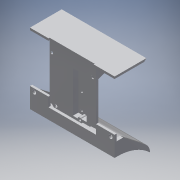
# Autodesk Inventor part: Chasis_base
Saved by Autodesk Inventor 2017 (Build 210142000, 142)
## iProperties
Created: 2018-02-27
Part Number: Chasis_base
Material: PAEK Plastic
Document SubType Name: Modeling
Designer: bradl
Density: 1.32 g/cm^3
Appearance: Smooth - White
Author: bradl
Autodesk Inventor part; units mm, degrees
ref_plane "YZ Plane" through (0, 0, 0) normal (1, 0, 0) x (0, 1, 0)
ref_plane "XZ Plane" through (0, 0, 0) normal (0, 1, 0) x (-1, 0, 0)
ref_plane "XY Plane" through (0, 0, 0) normal (0, 0, 1) x (1, 0, 0)
sketch "Sketch1" plane through (0, 0, 0) normal (0, 0, 1) x (1, 0, 0)
  arc A0 (-11.1125, -2.3813) -> (-3.175, -2.3812) centre (-7.1437, -2.3813) ccw projected
  arc A1 (5.2705, 38.0653) -> (-2.667, 38.0653) centre (1.3018, 38.0653) ccw projected
  line L0 (1.3018, 42.034) -> (-11.1125, 42.034)
  line L1 (-11.1125, 42.034) -> (-11.1125, -6.35)
  line L2 (-11.1125, -6.35) -> (5.2705, -6.35)
  line L3 (5.2705, -6.35) -> (5.2705, 42.034)
  line L4 (5.2705, 42.034) -> (1.3018, 42.034)
  circle A2 centre (-7.1437, -2.3813) radius 1.27 projected
  circle A3 centre (-7.1438, 16.9213) radius 1.27 projected
  circle A4 centre (1.3018, 18.7628) radius 1.27 projected
  circle A5 centre (1.3018, 38.0653) radius 1.27 projected
  circle A6 centre (-7.1437, -2.3813) radius 1.27
  circle A7 centre (-7.1438, 16.9213) radius 1.27
  circle A8 centre (1.3018, 18.7628) radius 1.27
  circle A9 centre (1.3018, 38.0653) radius 1.27
  point P0 (0, 0)
  constraints: 10 end point, 4 centre point, 4 coincident, 4 concentric, 4 perpendicular, 1 horizontal, 1 point on circle, 1 point on line, 1 tangent
extrude "Extrusion1" add sketch "Sketch1" along normal blind 2.54
sketch "Sketch2" plane through (0, 0, 2.54) normal (0, 0, 1) x (1, 0, 0)
  circle A0 centre (1.3018, 38.0653) radius 1.27 projected
  circle A1 centre (1.3018, 18.7628) radius 1.27 projected
  circle A2 centre (-7.1438, 16.9213) radius 1.27 projected
  circle A3 centre (-7.1437, -2.3813) radius 1.27 projected
  line L0 (5.2705, 42.034) -> (-11.1125, 42.034) projected
  line L1 (-11.1125, 42.034) -> (-11.1125, -6.35) projected
  line L2 (-11.1125, -6.35) -> (5.2705, -6.35) projected
  line L3 (5.2705, -6.35) -> (5.2705, 42.034) projected
  line L4 (-11.1125, -6.35) -> (5.2705, -6.35) projected
  line L5 (5.2705, -6.35) -> (5.2705, 42.034) projected
  line L6 (5.2705, -6.35) -> (5.2705, 42.034)
  line L7 (5.2705, 42.034) -> (-11.1125, 42.034) projected
  line L8 (5.2705, 42.034) -> (-11.1125, 42.034)
  line L9 (-11.1125, 42.034) -> (-11.1125, -6.35) projected
  line L10 (-11.1125, 42.034) -> (-11.1125, -6.35)
  line L11 (-11.1125, -6.35) -> (5.2705, -6.35)
  line L12 (5.2705, -6.35) -> (5.2705, -8.89) construction
  line L13 (-11.1125, -6.35) -> (-13.6525, -6.35) construction
  line L14 (5.2705, -8.89) -> (-13.6525, -8.89)
  line L15 (-11.1125, 42.034) -> (-11.1125, 44.574) construction
  line L16 (5.2705, 42.034) -> (7.8105, 42.034) construction
  line L17 (-13.6525, -8.89) -> (-13.6525, 44.574)
  line L18 (-13.6525, 44.574) -> (7.8105, 44.574)
  line L19 (7.8105, 44.574) -> (7.8105, -8.89)
  line L20 (7.8105, -8.89) -> (5.2705, -8.89)
  point P0 (0, 0)
  dimension "d2" = 2.54
  dimension "d3" = 2.54
  dimension "d4" = 2.54
  dimension "d5" = 2.54
  constraints: 26 end point, 4 collinear, 3 perpendicular, 2 horizontal, 2 point on line, 2 vertical
  measures "d2" distance of L2.end L12.end
  measures "d3" distance of L1.end L13.end
  measures "d4" distance of L0.end L15.end
  measures "d5" distance of L0.start L16.end
extrude "Extrusion2" add sketch "Sketch2" along normal blind 5.08 and the other way blind 2.54 contours L14 L17 L18 L19 L20
sketch "Sketch3" plane through (0, 0, 7.62) normal (0, 0, 1) x (1, 0, 0)
  line L0 (7.8105, -8.89) -> (7.8105, 44.574) projected
  line L1 (-13.6525, -8.89) -> (7.8105, -8.89) projected
  line L2 (-13.6525, 44.574) -> (-13.6525, -8.89) projected
  line L3 (7.8105, 44.574) -> (-13.6525, 44.574) projected
  line L4 (-13.6525, 44.574) -> (7.8105, 44.574) projected
  line L5 (7.8105, 44.574) -> (-13.6525, 44.574)
  line L6 (-13.6525, 44.574) -> (-13.6525, -8.89)
  line L7 (-13.6525, -8.89) -> (7.8105, -8.89)
  line L8 (7.8105, -8.89) -> (7.8105, 44.574)
  line L9 (20.033, 8.7532) -> (20.033, 11.6691) projected
  line L10 (-41.2425, 9.6344) -> (-41.2425, 7.0138) projected
  line L11 (20.033, 8.7532) -> (17.493, 8.7532) construction
  line L12 (-41.2425, 7.0138) -> (-38.7025, 7.0138) construction
  line L13 (17.493, 8.7532) -> (-38.7025, 8.7532) construction
  line L14 (17.493, 8.7532) -> (17.493, 59.5532) construction
  line L15 (17.493, 59.5532) -> (-38.7025, 59.5532) construction
  line L16 (-38.7025, 59.5532) -> (-38.7025, -39.5068) construction
  line L17 (-38.7025, -39.5068) -> (17.493, -39.5068) construction
  line L18 (17.493, -39.5068) -> (17.493, 8.7532) construction
  line L19 (17.493, 59.5532) -> (-38.7025, 59.5532)
  line L20 (-38.7025, 59.5532) -> (-38.7025, -39.5068)
  line L21 (-38.7025, -39.5068) -> (17.493, -39.5068)
  line L22 (17.493, -39.5068) -> (17.493, 59.5532)
  line L23 (-11.1125, 42.034) -> (5.2705, 42.034) projected
  line L24 (-11.1125, 42.034) -> (-11.1125, -6.35) projected
  line L25 (5.2705, 42.034) -> (-11.1125, 42.034)
  line L26 (-11.1125, 42.034) -> (-11.1125, -6.35)
  line L27 (-11.1125, -6.35) -> (5.2705, -6.35)
  line L28 (5.2705, -6.35) -> (5.2705, 42.034)
  point P0 (0, 0)
  dimension "d10" = 2.54
  dimension "d11" = 2.54
  dimension "d12" = 50.8
  dimension "d13" = 99.06
  constraints: 40 end point, 6 horizontal, 6 parallel, 6 perpendicular, 1 collinear, 1 point on line, 1 vertical
  measures "d10" distance of L9.start L11.end
  measures "d11" distance of L10.end L12.end
  measures "d12" distance of L11.end L14.end
  measures "d13" distance of L15.end L16.end
extrude "Extrusion3" add sketch "Sketch3" along normal blind 2.54 contours L1 L2 L3 L0 | L22 L21 L20 L19
sketch "Sketch4" plane through (0, 0, 7.62) normal (0, 0, -1) x (-1, 0, 0)
  line L0 (18.4925, 33.414) -> (14.6525, 33.414)
  line L1 (18.4925, 33.414) -> (18.4925, 23.414) projected
  line L2 (14.6525, 23.414) -> (14.6525, 33.414) projected
  line L3 (18.4925, 23.414) -> (14.6525, 23.414)
  line L4 (31.1925, 23.414) -> (31.1925, 33.414) projected
  line L5 (35.0325, 33.414) -> (31.1925, 33.414)
  line L6 (35.0325, 33.414) -> (35.0325, 23.414) projected
  line L7 (35.0325, 23.414) -> (31.1925, 23.414)
  line L8 (14.6525, 23.414) -> (18.4925, 23.414)
  line L9 (18.4925, 23.414) -> (18.4925, 33.414)
  line L10 (18.4925, 33.414) -> (14.6525, 33.414)
  line L11 (14.6525, 33.414) -> (14.6525, 23.414)
  line L12 (31.1925, 23.414) -> (35.0325, 23.414)
  line L13 (35.0325, 23.414) -> (35.0325, 33.414)
  line L14 (35.0325, 33.414) -> (31.1925, 33.414)
  line L15 (31.1925, 33.414) -> (31.1925, 23.414)
  point P0 (0, 0)
  constraints: 24 end point, 6 horizontal, 4 parallel, 2 perpendicular, 3 other
extrude "Extrusion4" add sketch "Sketch4" along normal blind 12.7
sketch "Sketch5" plane through (-35.0325, 23.414, 7.62) normal (-1, 0, 0) x (0, 0, 1)
  line L0 (0, 0) -> (-12.7, 0) projected
  line L1 (0, 10) -> (-12.7, 10) projected
  circle A0 centre (-12.7, 5.0827) radius 4.9173
  point P0 (-7.62, -23.414)
  constraints: 1 vertical alignment, 2 other
extrude "Extrusion5" cut sketch "Sketch5" against normal blind 20.6375
sketch "Sketch6" plane through (17.493, -39.5068, 7.62) normal (1, 0, 0) x (0, 0, -1)
  line L0 (0, 0) -> (0, 99.06) projected
  line L1 (0, 99.06) -> (0, 15.8755) construction
  line L2 (-13.9711, 65.9208) -> (-12.7011, 65.9208) construction
  arc A0 (-12.7011, 65.9208) -> (-12.403, 63.5609) centre (12.62, 67.9208) ccw construction
  line L3 (-12.403, 63.5609) -> (-13.6331, 63.245) construction
  line L4 (-13.6331, 63.245) -> (-12.6383, 59.3707) construction
  line L5 (-12.6383, 59.3707) -> (-11.4082, 59.6865) construction
  arc A1 (-11.4082, 59.6865) -> (-10.5326, 57.4749) centre (12.62, 67.9208) ccw construction
  line L6 (-10.5326, 57.4749) -> (-11.6455, 56.8631) construction
  line L7 (-11.6455, 56.8631) -> (-9.7185, 53.3578) construction
  line L8 (-9.7185, 53.3578) -> (-8.6056, 53.9697) construction
  arc A2 (-8.6056, 53.9697) -> (-7.2074, 52.0452) centre (12.62, 67.9208) ccw construction
  line L9 (-7.2074, 52.0452) -> (-8.1332, 51.1759) construction
  line L10 (-8.1332, 51.1759) -> (-5.395, 48.26) construction
  line L11 (-5.395, 48.26) -> (-4.4692, 49.1294) construction
  arc A3 (-4.4692, 49.1294) -> (-2.6364, 47.6131) centre (12.62, 67.9208) ccw construction
  line L12 (-2.6364, 47.6131) -> (-3.3169, 46.5408) construction
  line L13 (-3.3169, 46.5408) -> (0.0604, 44.3975) construction
  line L14 (0.0604, 44.3975) -> (0.7409, 45.4698) construction
  arc A4 (0.7409, 45.4698) -> (2.8932, 44.457) centre (12.62, 67.9208) ccw construction
  line L15 (2.8932, 44.457) -> (2.5008, 43.2492) construction
  line L16 (2.5008, 43.2492) -> (6.305, 42.0131) construction
  line L17 (6.305, 42.0131) -> (6.6975, 43.221) construction
  arc A5 (6.6975, 43.221) -> (9.034, 42.7752) centre (12.62, 67.9208) ccw construction
  line L18 (9.034, 42.7752) -> (8.9543, 41.5077) construction
  line L19 (8.9543, 41.5077) -> (12.9464, 41.2566) construction
  line L20 (12.9464, 41.2566) -> (13.0261, 42.5241) construction
  arc A6 (13.0261, 42.5241) -> (15.4001, 42.6734) centre (12.62, 67.9208) ccw construction
  line L21 (15.4001, 42.6734) -> (15.6381, 41.4259) construction
  line L22 (15.6381, 41.4259) -> (19.5673, 42.1755) construction
  line L23 (19.5673, 42.1755) -> (19.3293, 43.423) construction
  arc A7 (19.3293, 43.423) -> (21.5916, 44.158) centre (12.62, 67.9208) ccw construction
  line L24 (21.5916, 44.158) -> (22.1323, 43.0089) construction
  line L25 (22.1323, 43.0089) -> (25.7516, 44.712) construction
  line L26 (25.7516, 44.712) -> (25.2109, 45.8611) construction
  arc A8 (25.2109, 45.8611) -> (27.2193, 47.1357) centre (12.62, 67.9208) ccw construction
  line L27 (27.2193, 47.1357) -> (28.0288, 46.1572) construction
  line L28 (28.0288, 46.1572) -> (31.1109, 48.7068) construction
  line L29 (31.1109, 48.7068) -> (30.3013, 49.6854) construction
  arc A9 (30.3013, 49.6854) -> (31.9297, 51.4194) centre (12.62, 67.9208) ccw construction
  line L30 (31.9297, 51.4194) -> (32.9571, 50.6729) construction
  line L31 (32.9571, 50.6729) -> (35.3083, 53.909) construction
  line L32 (35.3083, 53.909) -> (34.2808, 54.6555) construction
  arc A10 (34.2808, 54.6555) -> (35.4267, 56.7399) centre (12.62, 67.9208) ccw construction
  line L33 (35.4267, 56.7399) -> (36.6076, 56.2724) construction
  line L34 (36.6076, 56.2724) -> (38.0801, 59.9915) construction
  line L35 (38.0801, 59.9915) -> (36.8992, 60.459) construction
  arc A11 (36.8992, 60.459) -> (37.4908, 62.763) centre (12.62, 67.9208) ccw construction
  line L36 (37.4908, 62.763) -> (38.7508, 62.6038) construction
  line L37 (38.7508, 62.6038) -> (39.2521, 66.5723) construction
  line L38 (39.2521, 66.5723) -> (37.9921, 66.7315) construction
  arc A12 (37.9921, 66.7315) -> (37.9921, 69.1102) centre (12.62, 67.9208) ccw construction
  line L39 (37.9921, 69.1102) -> (39.2521, 69.2693) construction
  line L40 (39.2521, 69.2693) -> (38.7508, 73.2378) construction
  line L41 (38.7508, 73.2378) -> (37.4908, 73.0786) construction
  arc A13 (37.4908, 73.0786) -> (36.8992, 75.3826) centre (12.62, 67.9208) ccw construction
  line L42 (36.8992, 75.3826) -> (38.0801, 75.8501) construction
  line L43 (38.0801, 75.8501) -> (36.6076, 79.5692) construction
  line L44 (36.6076, 79.5692) -> (35.4267, 79.1017) construction
  arc A14 (35.4267, 79.1017) -> (34.2808, 81.1862) centre (12.62, 67.9208) ccw construction
  line L45 (34.2808, 81.1862) -> (35.3083, 81.9327) construction
  line L46 (35.3083, 81.9327) -> (32.9571, 85.1687) construction
  line L47 (32.9571, 85.1687) -> (31.9297, 84.4222) construction
  arc A15 (31.9297, 84.4222) -> (30.3013, 86.1562) centre (12.62, 67.9208) ccw construction
  line L48 (30.3013, 86.1562) -> (31.1109, 87.1348) construction
  line L49 (31.1109, 87.1348) -> (28.0288, 89.6845) construction
  line L50 (28.0288, 89.6845) -> (27.2193, 88.7059) construction
  arc A16 (27.2193, 88.7059) -> (25.2109, 89.9805) centre (12.62, 67.9208) ccw construction
  line L51 (25.2109, 89.9805) -> (25.7516, 91.1296) construction
  line L52 (25.7516, 91.1296) -> (22.1323, 92.8328) construction
  line L53 (22.1323, 92.8328) -> (21.5916, 91.6836) construction
  arc A17 (21.5916, 91.6836) -> (19.3293, 92.4187) centre (12.62, 67.9208) ccw construction
  line L54 (19.3293, 92.4187) -> (19.5673, 93.6662) construction
  line L55 (19.5673, 93.6662) -> (15.6381, 94.4157) construction
  line L56 (15.6381, 94.4157) -> (15.4001, 93.1682) construction
  arc A18 (15.4001, 93.1682) -> (13.0261, 93.3176) centre (12.62, 67.9208) ccw construction
  line L57 (13.0261, 93.3176) -> (12.9464, 94.5851) construction
  line L58 (12.9464, 94.5851) -> (8.9543, 94.3339) construction
  line L59 (8.9543, 94.3339) -> (9.034, 93.0664) construction
  arc A19 (9.034, 93.0664) -> (6.6975, 92.6207) centre (12.62, 67.9208) ccw construction
  line L60 (6.6975, 92.6207) -> (6.305, 93.8285) construction
  line L61 (6.305, 93.8285) -> (2.5008, 92.5925) construction
  line L62 (2.5008, 92.5925) -> (2.8932, 91.3846) construction
  arc A20 (2.8932, 91.3846) -> (0.7409, 90.3718) centre (12.62, 67.9208) ccw construction
  line L63 (0.7409, 90.3718) -> (0.0604, 91.4441) construction
  line L64 (0.0604, 91.4441) -> (-3.3169, 89.3008) construction
  line L65 (-3.3169, 89.3008) -> (-2.6364, 88.2285) construction
  arc A21 (-2.6364, 88.2285) -> (-4.4692, 86.7123) centre (12.62, 67.9208) ccw construction
  line L66 (-4.4692, 86.7123) -> (-5.395, 87.5816) construction
  line L67 (-5.395, 87.5816) -> (-8.1332, 84.6658) construction
  line L68 (-8.1332, 84.6658) -> (-7.2074, 83.7964) construction
  arc A22 (-7.2074, 83.7964) -> (-8.6056, 81.872) centre (12.62, 67.9208) ccw construction
  line L69 (-8.6056, 81.872) -> (-9.7185, 82.4838) construction
  line L70 (-9.7185, 82.4838) -> (-11.6455, 78.9786) construction
  line L71 (-11.6455, 78.9786) -> (-10.5326, 78.3668) construction
  arc A23 (-10.5326, 78.3668) -> (-11.4082, 76.1551) centre (12.62, 67.9208) ccw construction
  line L72 (-11.4082, 76.1551) -> (-12.6383, 76.4709) construction
  line L73 (-12.6383, 76.4709) -> (-13.6331, 72.5966) construction
  line L74 (-13.6331, 72.5966) -> (-12.403, 72.2808) construction
  arc A24 (-12.403, 72.2808) -> (-12.7011, 69.9208) centre (12.62, 67.9208) ccw construction
  line L75 (-12.7011, 69.9208) -> (-13.9711, 69.9208) construction
  line L76 (-13.9711, 69.9208) -> (-13.9711, 65.9208) construction
  circle A25 centre (12.62, 67.9208) radius 21.59 construction
  circle A26 centre (12.62, 67.9208) radius 26.6867 construction
  line L77 (0, 99.06) -> (39.3067, 99.06) construction
  line L78 (39.3067, 99.06) -> (39.3067, 0.6575) construction
  arc A27 (39.3067, 0.6575) -> (0, 15.8755) centre (0.9026, -40.1652) ccw
  line L79 (39.3067, 0.6575) -> (39.3067, 7.6204)
  line L80 (39.3067, 0.6575) -> (46.2696, 0.6575) construction
  line L81 (0, 99.06) -> (0, 0) projected
  arc A28 (39.3067, 7.6204) -> (0, 20.9929) centre (1.7012, -38.4614) ccw
  line L82 (0, 20.9929) -> (0, 15.8755)
  line L83 (0, 20.9929) -> (5.1174, 20.9929) construction
  point P0 (7.62, 39.5068)
  dimension "d20" = 90
  dimension "d21" = 90
  dimension "d22" = 90
  constraints: 14 end point, 4 point on circle, 3 centre point, 3 horizontal, 2 perpendicular, 2 point on line, 1 coincident, 1 vertical
  measures "d20" angle of L77 L78
  measures "d21" angle of L80 L79
  measures "d22" angle of L82 L83
extrude "Extrusion6" add sketch "Sketch6" against normal blind 56.1848
sketch "Sketch7" plane through (-38.7025, -39.5068, 7.62) normal (-1, 0, 0) x (0, 0, 1)
  arc A0 (0, 15.8755) -> (-39.3067, 0.6575) centre (-0.9026, -40.1652) ccw projected
  line L0 (0, 99.06) -> (0, 0) projected
  line L1 (0, 0) -> (2.54, 0) projected
  line L2 (2.54, 99.06) -> (2.54, 0) projected
  line L3 (0, 99.06) -> (2.54, 99.06) projected
  line L4 (0, 15.8755) -> (0, 0)
  line L5 (0, 0) -> (2.54, 0) projected
  line L6 (2.54, 0) -> (2.54, 15.8755)
  line L7 (2.54, 0) -> (2.54, 99.06) projected
  line L8 (0, 15.8755) -> (2.54, 15.8755)
  line L9 (0, 0) -> (2.54, 0)
  point P0 (-7.62, 39.5068)
  constraints: 8 end point, 1 horizontal, 1 parallel, 1 point on line, 1 vertical
extrude "Extrusion7" cut sketch "Sketch7" against normal blind 62.5348 contours L8 L2 L1 L0
sketch "Sketch8" plane through (17.493, -18.5139, 7.62) normal (1, 0, 0) x (0, 0, -1)
  line L0 (-2.54, -5.1174) -> (0, -5.1174) projected
  arc A0 (39.3067, -20.3354) -> (0, -5.1174) centre (0.9026, -61.1581) ccw projected
  line L1 (39.3067, -20.3354) -> (39.3067, -13.3725) projected
  arc A1 (39.3067, -13.3725) -> (0, 0) centre (1.7012, -59.4543) ccw projected
  line L2 (0, 0) -> (0, 78.0671) projected
  line L3 (0, 78.0671) -> (-2.54, 78.0671) projected
  line L4 (-2.54, -5.1174) -> (-2.54, 78.0671) projected
  arc A2 (39.3067, -20.3354) -> (0, -5.1174) centre (0.9026, -61.1581) ccw projected
  arc A3 (0, -5.1174) -> (0, -5.1174) centre (0, -61.1653) ccw
  arc A4 (39.3067, -13.3725) -> (0, 0) centre (1.7012, -59.4543) ccw
  arc A5 (39.3067, -20.3354) -> (0, -5.1174) centre (0.9026, -61.1581) ccw
  line L5 (0, -5.1174) -> (-2.54, -5.1174)
  line L6 (-2.54, -5.1174) -> (-2.54, 78.0671) projected
  line L7 (-2.54, 18.5139) -> (0, 18.5139)
  line L8 (39.3067, -20.3354) -> (39.3067, -13.3725)
  line L9 (-2.54, -5.1174) -> (-2.54, 18.5139)
  line L10 (0, 0) -> (0, 78.0671) projected
  line L11 (0, 18.5139) -> (0, 0)
  point P0 (7.62, 18.5139)
  constraints: 10 end point, 4 point on circle, 2 centre point, 2 horizontal, 2 point on line, 2 vertical, 1 collinear, 1 perpendicular, 1 vertical alignment, 3 other
extrude "Extrusion8" add sketch "Sketch8" along normal blind 21.844 and the other way blind 78.0288 contours L4 L7 L2 A1 L1 A0 L0
fillet "Fillet2" radius 14.2875 1 edges at (-10.5994, -31.8864, -31.6867)
sketch "Sketch9" plane through (39.337, -18.5139, 7.62) normal (1, 0, 0) x (0, 0, -1)
  arc A0 (39.3067, -20.3354) -> (32.3992, -8.5098) centre (25.0251, -20.7473) ccw projected
  arc A1 (32.3992, -8.5098) -> (0, 0) centre (1.7012, -59.4543) ccw projected
  line L0 (0, 0) -> (0, 18.5139) projected
  line L1 (0, 18.5139) -> (-2.54, 18.5139) projected
  line L2 (-2.54, 18.5139) -> (-2.54, -5.1174) projected
  line L3 (-2.54, -5.1174) -> (0, -5.1174) projected
  arc A2 (39.3067, -20.3354) -> (0, -5.1174) centre (0.9026, -61.1581) ccw projected
  arc A3 (39.3067, -20.3354) -> (0, -5.1174) centre (0.9026, -61.1581) ccw
  line L4 (0, -5.1174) -> (-2.54, -5.1174)
  line L5 (-2.54, -5.1174) -> (-2.54, 18.5139)
  line L6 (-2.54, 78.0671) -> (-2.54, 18.5139) projected
  line L7 (-2.54, 18.5139) -> (32.4002, -8.5104)
  arc A4 (32.3992, -8.5098) -> (0, 0) centre (1.7012, -59.4543) ccw projected
  line L8 (-2.54, 18.5139) -> (41.6316, 18.5139) construction
  line L9 (32.4002, -8.5104) -> (39.3067, -20.3354)
  point P0 (7.62, 18.5139)
  dimension "d33" = 37.72
  constraints: 10 end point, 3 point on circle, 2 horizontal, 1 centre point, 1 collinear, 1 equal length
  measures "d33" angle of L7 L8
extrude "Extrusion9" add sketch "Sketch9" against normal blind 3.81 contours A2 L3 L2 L7 L0 A1 L9 | A1 L0 L7
sketch "Sketch10" plane through (-60.5358, -18.5139, 7.62) normal (-1, 0, 0) x (0, 0, 1)
  arc A0 (-32.3992, -8.5098) -> (-39.3067, -20.3354) centre (-25.0251, -20.7473) ccw projected
  arc A1 (0, -5.1174) -> (-39.3067, -20.3354) centre (-0.9026, -61.1581) ccw projected
  line L0 (0, -5.1174) -> (2.54, -5.1174) projected
  line L1 (2.54, -5.1174) -> (2.54, 18.5139) projected
  line L2 (2.54, 18.5139) -> (0, 18.5139) projected
  line L3 (0, 18.5139) -> (0, 0) projected
  arc A2 (0, 0) -> (-32.3992, -8.5098) centre (-1.7012, -59.4543) ccw projected
  arc A3 (0, -5.1174) -> (-39.3067, -20.3354) centre (-0.9026, -61.1581) ccw projected
  arc A4 (0, -5.1174) -> (-39.3067, -20.3354) centre (-0.9026, -61.1581) ccw
  line L4 (2.54, -5.1174) -> (0, -5.1174) projected
  line L5 (0, -5.1174) -> (2.54, -5.1174)
  line L6 (2.54, 18.5139) -> (2.54, -5.1174) projected
  line L7 (2.54, -5.1174) -> (2.54, 18.5139)
  arc A5 (0, 0) -> (-32.3992, -8.5098) centre (-1.7012, -59.4543) ccw projected
  line L8 (2.54, 18.5139) -> (-32.3992, -8.5098)
  line L9 (-32.3992, -8.5098) -> (-39.3067, -20.3354)
  point P0 (-7.62, 18.5139)
  constraints: 8 end point, 2 point on circle, 1 centre point, 1 horizontal, 1 perpendicular
extrude "Extrusion10" add sketch "Sketch10" against normal blind 3.81 contours L8 L3 A2 | A2 L3 L8 L1 L0 A1 L9
sketch "Sketch12" plane through (0, 0, 2.54) normal (0, 0, 1) x (1, 0, 0)
  circle A0 centre (1.3018, 38.0653) radius 1.27 projected
  circle A1 centre (1.3018, 18.7628) radius 1.27 projected
  circle A2 centre (-7.1438, 16.9213) radius 1.27 projected
  circle A3 centre (-7.1437, -2.3813) radius 1.27 projected
  line L0 (5.2705, 42.034) -> (-11.1125, 42.034) projected
  line L1 (-11.1125, 42.034) -> (-11.1125, -6.35) projected
  line L2 (-11.1125, -6.35) -> (5.2705, -6.35) projected
  line L3 (5.2705, -6.35) -> (5.2705, 42.034) projected
  line L4 (-11.1125, 42.034) -> (5.2705, 42.034) projected
  line L5 (17.493, 0) -> (39.337, 0) projected
  line L6 (-11.1125, 0) -> (-11.1125, 42.034) projected
  line L7 (39.337, -23.6314) -> (-60.5358, -23.6314) projected
  line L8 (39.337, 0) -> (39.337, -23.6314) projected
  line L9 (17.493, 0) -> (17.493, 59.5532) projected
  line L10 (17.493, 59.5532) -> (-38.7025, 59.5532) projected
  line L11 (-38.7025, 59.5532) -> (-38.7025, 0) projected
  line L12 (-60.5358, 0) -> (-38.7025, 0) projected
  line L13 (-60.5358, -23.6314) -> (-60.5358, 0) projected
  line L14 (5.2705, -6.35) -> (5.2705, 0) projected
  line L15 (-11.1125, 0) -> (5.2705, 0)
  line L16 (5.2705, 0) -> (5.2705, -6.35)
  line L17 (5.2705, -6.35) -> (-11.1125, -6.35)
  line L18 (-11.1125, -6.35) -> (-11.1125, 0)
  line L19 (5.2705, 42.034) -> (5.2705, 0) projected
  line L20 (-11.1125, 0) -> (5.2705, 0) projected
  point P0 (0, 0)
  constraints: 8 end point, 2 parallel, 1 horizontal, 1 perpendicular
extrude "Extrusion12" cut sketch "Sketch12" along normal blind 14.9225 contours A3 | L3 L2 L1 L15
sketch "Sketch13" plane through (0, 0, 10.16) normal (0, 0, 1) x (1, 0, 0)
  line L0 (-38.7025, 59.5532) -> (14.6375, 59.5532) projected
  line L1 (-38.7025, -6.4868) -> (-38.7025, 59.5532) projected
  line L2 (-36.226, -6.4868) -> (-38.7025, -6.4868) projected
  line L3 (-33.6225, -9.0268) -> (-36.1176, -6.5317) projected
  line L4 (-0.8565, -9.0268) -> (-33.6225, -9.0268) projected
  line L5 (1.6386, -6.5317) -> (-0.8565, -9.0268) projected
  line L6 (13.1135, -6.4868) -> (1.747, -6.4868) projected
  line L7 (14.6375, 59.5532) -> (14.6375, -4.9628) projected
  line L8 (14.6375, -4.9628) -> (13.1135, -6.4868) projected
  line L9 (17.493, 59.5532) -> (-38.7025, 59.5532) projected
  line L10 (-38.7025, 59.5532) -> (14.6375, 59.5532)
  line L11 (14.6375, -4.9628) -> (13.1135, -6.4868)
  line L12 (14.6375, -4.9628) -> (14.6375, 59.5532)
  line L13 (13.1135, -6.4868) -> (1.747, -6.4868)
  line L14 (-11.1125, -6.35) -> (5.2705, -6.35) projected
  line L15 (-0.8565, -9.0268) -> (1.747, -6.4868)
  line L16 (-0.8565, -9.0268) -> (-33.6225, -9.0268)
  line L17 (-36.1176, -6.5317) -> (-33.6225, -9.0268)
  line L18 (-36.1176, -6.5317) -> (-38.7025, -6.4868)
  line L19 (-38.7025, -6.4868) -> (-38.7025, 59.5532)
  point P0 (0, 0)
  constraints: 18 end point, 2 collinear, 2 perpendicular, 1 parallel
extrude "Extrusion13" cut sketch "Sketch13" against normal blind 1.27
sketch "Sketch14" plane through (0, 0, 10.16) normal (0, 0, 1) x (1, 0, 0)
  line L0 (14.6375, 59.5532) -> (14.6375, -4.9628) projected
  line L1 (14.6375, -4.9628) -> (13.1135, -6.4868) projected
  line L2 (13.1135, -6.4868) -> (1.747, -6.4868) projected
  line L3 (1.747, -6.4868) -> (-0.8565, -9.0268) projected
  line L4 (-0.8565, -9.0268) -> (-33.6225, -9.0268) projected
  line L5 (-33.6225, -9.0268) -> (-36.1176, -6.5317) projected
  line L6 (-36.1176, -6.5317) -> (-38.7025, -6.4868) projected
  line L7 (-38.7025, -6.4868) -> (-38.7025, 0) projected
  line L8 (-60.5358, 0) -> (-38.7025, 0) projected
  line L9 (-60.5358, -23.6314) -> (-60.5358, 0) projected
  line L10 (39.337, -23.6314) -> (-60.5358, -23.6314) projected
  line L11 (39.337, 0) -> (39.337, -23.6314) projected
  line L12 (17.493, 0) -> (39.337, 0) projected
  line L13 (17.493, 0) -> (17.493, 59.5532) projected
  line L14 (17.493, 59.5532) -> (14.6375, 59.5532) projected
  line L15 (-36.1176, -6.5317) -> (-38.7025, -6.4868) projected
  line L16 (-38.7025, -6.4868) -> (-36.1176, -6.5317)
  line L17 (-33.6225, -9.0268) -> (-36.1176, -6.5317) projected
  line L18 (-36.1176, -6.5317) -> (-33.6225, -9.0268)
  line L19 (-33.6225, -9.0268) -> (-0.8565, -9.0268)
  line L20 (7.8105, -8.89) -> (-13.6525, -8.89) projected
  line L21 (1.747, -6.4868) -> (-0.8565, -9.0268) projected
  line L22 (13.1135, -6.4868) -> (1.747, -6.4868) projected
  line L23 (1.747, -6.4868) -> (13.1135, -6.4868)
  line L24 (14.6375, 59.5532) -> (14.6375, -4.9628) projected
  line L25 (13.1135, -6.4868) -> (14.6375, -4.9628)
  line L26 (14.6375, -4.9628) -> (17.493, -4.9628)
  line L27 (17.493, -4.9628) -> (17.493, -10.8663)
  line L28 (-38.7025, -6.4868) -> (-38.7025, -10.8663)
  line L29 (-38.7025, -10.8663) -> (17.493, -10.8663)
  point P0 (0, 0)
  constraints: 18 end point, 3 perpendicular, 2 parallel, 1 collinear, 1 horizontal, 1 vertical
extrude "Extrusion14" cut sketch "Sketch14" against normal blind 2.54 contours L26 L27 L29 L28 L6 L5 L4 L3 L2 L1
sketch "Sketch15" plane through (0, 0, 7.62) normal (0, 0, -1) x (-1, 0, 0)
  line L0 (-17.493, 59.5532) -> (38.7025, 59.5532) projected
  line L1 (38.7025, 59.5532) -> (38.7025, 0) projected
  line L2 (-17.493, 0) -> (-17.493, 59.5532) projected
  line L3 (60.5465, 52.8441) -> (60.5465, 51.6457) projected
  line L4 (-39.337, 50.4737) -> (-39.337, 51.6228) projected
  line L5 (60.5465, 59.5532) -> (-39.337, 59.5532)
  line L6 (-39.337, 59.5532) -> (-39.337, 57.0132)
  line L7 (-39.337, 57.0132) -> (60.5465, 57.0132)
  line L8 (60.5465, 57.0132) -> (60.5465, 59.5532)
  point P0 (0, 0)
  dimension "d47" = 2.54
  constraints: 8 end point, 2 parallel, 1 horizontal, 1 perpendicular
  measures "d47" distance of L6.end L5.end
extrude "Extrusion15" add sketch "Sketch15" along normal blind 34.925
chamfer "Chamfer1" distance 2.54 angle 45 1 edges at (-10.6047, 57.0132, -27.305)
sketch "Sketch16" plane through (-38.7025, 0, 8.89) normal (-1, 0, 0) x (0, 0, 1)
  line L0 (-1.27, 44.574) -> (-8.89, 44.574) projected
  line L1 (-1.27, 57.0132) -> (-33.655, 57.0132) projected
  line L2 (-1.27, 44.574) -> (-33.655, 57.0132)
  line L3 (-1.27, 57.0132) -> (-3.81, 57.0132) projected
  line L4 (-33.655, 57.0132) -> (-1.27, 57.0132)
  line L5 (-1.27, 57.0132) -> (-1.27, 44.574)
  point P0 (-8.89, 0)
  constraints: 6 end point, 1 horizontal, 1 perpendicular
extrude "Extrusion16" add sketch "Sketch16" against normal blind 2.54
sketch "Sketch17" plane through (17.493, 0, 10.16) normal (1, 0, 0) x (0, 0, -1)
  line L0 (2.54, 44.574) -> (10.16, 44.574) projected
  line L1 (2.54, 44.574) -> (34.925, 57.0132) projected
  line L2 (2.54, 57.0132) -> (34.925, 57.0132) projected
  line L3 (2.54, 57.0132) -> (5.08, 57.0132) projected
  line L4 (2.54, 0) -> (2.54, 57.0132) projected
  line L5 (2.54, 44.574) -> (2.54, 57.0132)
  line L6 (34.925, 57.0132) -> (2.54, 57.0132)
  line L7 (34.925, 57.0132) -> (2.54, 44.574)
  point P0 (10.16, 0)
  constraints: 6 end point, 2 collinear, 1 vertical
extrude "Extrusion17" add sketch "Sketch17" against normal blind 2.54
sketch "Sketch18" plane through (0, 0, 10.16) normal (0, 0, 1) x (1, 0, 0)
  circle A0 centre (-31.0825, -6.4868) radius 1.6 projected
  circle A1 centre (-3.1425, -6.4868) radius 1.6 projected
  circle A2 centre (12.0975, 44.3132) radius 1.6 projected
  circle A3 centre (-36.1625, 45.5832) radius 1.6 projected
  circle A4 centre (-31.0825, -6.4868) radius 1.6
  circle A5 centre (-3.1425, -6.4868) radius 1.6
  circle A6 centre (12.0975, 44.3132) radius 1.6
  circle A7 centre (-36.1625, 45.5832) radius 1.6
  point P0 (0, 0)
  constraints: 4 centre point, 4 coincident, 3 concentric
extrude "Extrusion18" cut sketch "Sketch18" against normal blind 25.4
sketch "Sketch19" plane through (-38.7025, 0, 8.89) normal (-1, 0, 0) x (0, 0, 1)
  line L0 (-1.27, 47.1832) -> (-1.27, 57.0132) projected
  line L1 (-1.27, 43.9832) -> (-1.27, 47.1832) projected
  line L2 (-33.655, 57.0132) -> (-1.27, 44.574) projected
  line L3 (-1.27, 49.0281) -> (-1.27, 44.574)
  line L4 (-1.27, 49.0281) -> (-12.8661, 49.0281)
  line L5 (-1.27, 44.574) -> (-8.0629, 47.1832) projected
  line L6 (-1.27, 44.574) -> (-12.8661, 49.0281)
  point P0 (-8.89, 0)
  constraints: 6 end point, 2 collinear, 2 point on line, 1 horizontal
extrude "Extrusion19" cut sketch "Sketch19" against normal blind 25.4
sketch "Sketch20" plane through (-14.6525, 23.414, 7.62) normal (1, 0, 0) x (0, 0, -1)
  arc A0 (12.7, 10) -> (12.7, 0.1653) centre (12.7, 5.0827) ccw projected
  line L0 (12.7, 0.1653) -> (12.7, 0)
  line L1 (12.7, 0) -> (12.7, 10)
  line L2 (12.7, 10) -> (11.6676, 10)
  line L3 (0, 10) -> (12.7, 10) projected
  line L4 (0, 0) -> (12.7, 0) projected
  line L5 (11.6676, 0) -> (12.7, 0)
  line L6 (12.7, 0) -> (11.6676, 0)
  line L7 (11.6676, 10) -> (11.6676, 0)
  point P0 (7.62, -23.414)
  constraints: 12 end point, 3 point on line, 2 collinear, 1 perpendicular, 1 vertical
extrude "Extrusion20" cut sketch "Sketch20" against normal blind 25.4 contours L1 A0 L7 | A0 L7 L2 | L0 L4 L7 A0
sketch "Sketch21" plane through (0, 0, 7.62) normal (0, 0, 1) x (1, 0, 0)
  line L0 (17.493, 59.5532) -> (39.337, 59.5532) projected
  line L1 (39.337, 57.0132) -> (17.493, 57.0132)
  line L2 (17.493, 57.0132) -> (17.493, 59.5532)
  line L3 (17.493, 59.5532) -> (39.337, 59.5532)
  line L4 (39.337, 59.5532) -> (39.337, 57.0132)
  line L5 (-60.5465, 59.5532) -> (-38.7025, 59.5532) projected
  line L6 (-38.7025, 57.0132) -> (-60.5465, 57.0132)
  line L7 (-60.5465, 57.0132) -> (-60.5465, 59.5532)
  line L8 (-60.5465, 59.5532) -> (-38.7025, 59.5532)
  line L9 (-38.7025, 59.5532) -> (-38.7025, 57.0132)
  point P0 (0, 0)
  constraints: 16 end point, 4 parallel, 2 horizontal, 2 perpendicular
extrude "Extrusion21" add sketch "Sketch21" along normal blind 2.54
sketch "Sketch22" plane through (0, 0, 10.16) normal (0, 0, 1) x (1, 0, 0)
  circle A0 centre (-55.5738, -3.9625) radius 2.286 projected
  line L0 (35.527, -1.9646) -> (35.527, -18.5139) projected
  circle A1 centre (34.6114, -4.2416) radius 2.286 projected
  circle A2 centre (-55.5738, -3.9625) radius 2.286
  circle A3 centre (34.6114, -4.2416) radius 2.286
  point P0 (0, 0)
  dimension "d68" = 4.572
  constraints: 2 centre point, 2 coincident, 1 concentric
  measures "d68" diameter of A3
extrude "Extrusion22" cut sketch "Sketch22" against normal blind 25.4
sketch "Sketch23" plane through (39.337, -18.5139, 7.62) normal (1, 0, 0) x (0, 0, -1)
  line L0 (0, 16.5494) -> (0, 18.5139) projected
  line L1 (0, 18.5139) -> (-2.54, 18.5139) projected
  line L2 (-2.54, 18.5139) -> (-2.54, -5.1174) projected
  line L3 (-2.54, -5.1174) -> (0, -5.1174) projected
  arc A0 (39.3067, -20.3354) -> (0, -5.1174) centre (0.9026, -61.1581) ccw projected
  arc A1 (39.3067, -20.3354) -> (32.4002, -8.5104) centre (25.0251, -20.7473) ccw projected
  line L4 (32.4002, -8.5104) -> (0, 16.5494) projected
  line L5 (32.3992, -8.5098) -> (5.136, 12.5769) projected
  line L6 (0, 16.5494) -> (7.62, 16.5494)
  line L7 (7.62, 16.5494) -> (7.62, 10.6557)
  line L8 (7.62, 10.6557) -> (0, 10.6557)
  line L9 (0, 10.6557) -> (0, 16.5494)
  point P0 (7.62, 18.5139)
  constraints: 8 end point, 2 parallel, 1 horizontal, 1 perpendicular, 1 point on line
extrude "Extrusion23" cut sketch "Sketch23" against normal blind 11.1125 contours L6 L7 L4 | L4 L8 L9
sketch "Sketch24" plane through (-60.5358, -18.5139, 7.62) normal (-1, 0, 0) x (0, 0, 1)
  line L0 (0, 9.6239) -> (-7.62, 9.6239) projected
  line L1 (0, 10.6557) -> (-7.62, 10.6557) projected
  line L2 (0, 10.6557) -> (-7.62, 10.6557)
  line L3 (0, 16.5494) -> (-32.3992, -8.5098) projected
  line L4 (0, 16.5494) -> (-7.62, 10.6557)
  line L5 (0, 16.526) -> (0, 10.6557)
  line L6 (0, 12.2654) -> (0, 16.8374) projected
  point P0 (-7.62, 18.5139)
  point P1 (0, 12.5769)
  constraints: 6 end point, 2 collinear, 1 horizontal
extrude "Extrusion24" cut sketch "Sketch24" against normal blind 25.4
sketch "Sketch25" plane through (0, 0, 8.89) normal (0, 0, 1) x (1, 0, 0)
  circle A0 centre (-3.1425, -6.4868) radius 1.6 projected
  circle A1 centre (-3.1425, -6.4868) radius 2.4134
  arc A2 (-4.7366, -6.35) -> (-1.5484, -6.35) centre (-3.1425, -6.4868) ccw projected
  circle A3 centre (-3.1425, -6.4868) radius 1.6
  point P0 (0, 0)
  constraints: 2 centre point, 2 coincident
extrude "Extrusion25" add sketch "Sketch25" against normal blind 7.9375
sketch "Sketch26" plane through (0, 0, 8.89) normal (0, 0, 1) x (1, 0, 0)
  circle A0 centre (-3.1425, -6.4868) radius 1.6 projected
  line L0 (-38.7025, -6.4868) -> (-38.7025, 0) projected
  line L1 (-36.1176, -6.5317) -> (-38.7025, -6.4868) projected
  line L2 (-33.6225, -9.0268) -> (-36.1176, -6.5317) projected
  line L3 (-0.8565, -9.0268) -> (-33.6225, -9.0268) projected
  line L4 (1.747, -6.4868) -> (-0.8565, -9.0268) projected
  line L5 (13.1135, -6.4868) -> (1.747, -6.4868) projected
  line L6 (14.6375, -4.9628) -> (13.1135, -6.4868) projected
  line L7 (14.6375, 59.5532) -> (14.6375, -4.9628) projected
  line L8 (-38.7025, 59.5532) -> (14.6375, 59.5532) projected
  line L9 (-38.7025, 57.0132) -> (-38.7025, 59.5532) projected
  line L10 (-38.7025, 0) -> (-38.7025, 57.0132) projected
  circle A1 centre (-36.1625, 45.5832) radius 1.6 projected
  circle A2 centre (-31.0825, -6.4868) radius 1.6 projected
  circle A3 centre (12.0975, 44.3132) radius 1.6 projected
  arc A4 (-0.733, -6.35) -> (-5.552, -6.35) centre (-3.1425, -6.4868) ccw projected
  line L11 (-11.1125, -6.35) -> (-5.552, -6.35) projected
  line L12 (-11.1125, 42.034) -> (-11.1125, -6.35) projected
  line L13 (5.2705, 42.034) -> (-11.1125, 42.034) projected
  line L14 (5.2705, -6.35) -> (5.2705, 42.034) projected
  line L15 (-0.733, -6.35) -> (5.2705, -6.35) projected
  arc A5 (-0.733, -6.35) -> (-5.552, -6.35) centre (-3.1425, -6.4868) ccw projected
  line L16 (5.2705, -6.35) -> (-1.4404, -6.35)
  line L17 (-1.4404, -6.35) -> (-1.4404, -4.7759)
  line L18 (-1.4404, -4.7759) -> (5.2705, -4.7759)
  line L19 (5.2705, -4.7759) -> (5.2705, -6.35)
  line L20 (5.2705, -4.7759) -> (-1.4404, -4.7759)
  line L21 (-1.4404, -4.7759) -> (-1.4404, -6.35)
  line L22 (-1.4404, -6.35) -> (5.2705, -6.35)
  line L23 (5.2705, -6.35) -> (5.2705, -4.7759)
  point P0 (0, 0)
  constraints: 16 end point, 4 parallel, 2 horizontal, 2 perpendicular, 2 point on circle
extrude "Extrusion26" add sketch "Sketch26" against normal blind 7.9375 contours A4 L18 L14 L15
sketch "Sketch27" plane through (-14.6525, 23.414, 7.62) normal (1, 0, 0) x (0, 0, -1)
  line L0 (0, 0) -> (11.6676, 0) projected
  line L1 (11.6676, 10.0141) -> (10.949, 10.0141)
  line L2 (10.949, 10.0141) -> (10.949, 0)
  line L3 (10.949, 0) -> (11.6676, 0)
  line L4 (11.6676, 0) -> (11.6676, 10.0141)
  point P0 (7.62, -23.414)
  constraints: 8 end point, 2 parallel, 1 horizontal, 1 perpendicular, 1 point on line
extrude "Extrusion27" cut sketch "Sketch27" against normal blind 25.4
body "Solid1"
